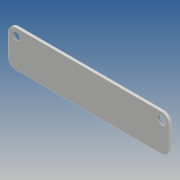
# Autodesk Inventor part: Light sensor ball guard
Saved by Autodesk Inventor 2017 (Build 210142000, 142)
## iProperties
Created: 2017-07-08
Part Number: Light sensor ball guard
Material: Generic
Document SubType Name: Modeling
Designer: yella
Density: 1 g/cm^3
Appearance: Default
Author: yella
Autodesk Inventor part; units mm, degrees
ref_plane "YZ Plane" through (0, 0, 0) normal (1, 0, 0) x (0, 1, 0)
ref_plane "XZ Plane" through (0, 0, 0) normal (0, 1, 0) x (-1, 0, 0)
ref_plane "XY Plane" through (0, 0, 0) normal (0, 0, 1) x (1, 0, 0)
sketch "Sketch1" plane through (0, 0, 0) normal (0, 1, 0) x (-1, 0, 0)
  circle A0 centre (28.2679, -64.7457) radius 1.6
  circle A1 centre (-28.2679, -64.7457) radius 1.6
  arc A2 (31.2679, -64.7457) -> (28.2679, -61.7457) centre (28.2679, -64.7457) ccw
  arc A3 (-28.2679, -61.7457) -> (-31.2679, -64.7457) centre (-28.2679, -64.7457) ccw
  line L0 (-28.2679, -61.7457) -> (28.2679, -61.7457)
  line L1 (48.3297, -88.9468) -> (2.1402, -66.9602)
  line L2 (-2.1585, -66.9605) -> (-48.3297, -88.9468)
  arc A4 (2.1402, -66.9602) -> (-2.1585, -66.9605) centre (-0.0088, -71.4748) ccw
  line L3 (-0.0092, -65.9371) -> (-0.0092, -75.9371)
  line L4 (-0.0092, -75.9371) -> (28.2679, -75.9371)
  line L5 (-0.0092, -75.9371) -> (-28.2679, -75.9371)
  line L6 (-31.2679, -72.9371) -> (-31.2679, -64.7457)
  line L7 (31.2679, -64.7457) -> (31.2679, -72.9371)
  arc A5 (28.2679, -75.9371) -> (31.2679, -72.9371) centre (28.2679, -72.9371) ccw
  arc A6 (-31.2679, -72.9371) -> (-28.2679, -75.9371) centre (-28.2679, -72.9371) ccw
  point P0 (0, 0)
  dimension "d0" = 3.2
  dimension "d1" = 3
  dimension "d2" = 3
  dimension "d3" = 5
  dimension "d4" = 10
  dimension "d5" = 3
  constraints: 16 end point, 10 point on circle, 7 centre point, 7 tangent, 2 coincident, 2 horizontal, 2 perpendicular, 1 equal radius, 1 parallel, 1 vertical
  measures "d0" diameter of A1
  measures "d1" radius of A2
  measures "d2" radius of A3
  measures "d3" radius of A4
  measures "d4" distance of L3.start L3.end
  measures "d5" radius of A5
extrude "Extrusion1" add sketch "Sketch1" along normal blind 1
body "Solid1"
